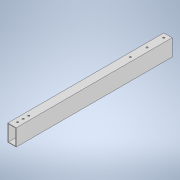
# Autodesk Inventor part: アーム3_角柱1
Saved by Autodesk Inventor 2021 (Build 250183000, 183)
## iProperties
Created: 2022-02-03
Part Number: アーム3_角柱1
Material: 一般
Document SubType Name: Modeling
Designer: hirohumi
Density: 1 g/cm^3
Appearance: 既定
Author: hirohumi
Autodesk Inventor part; units mm, degrees
ref_plane "YZ Plane" through (0, 0, 0) normal (1, 0, 0) x (0, 1, 0)
ref_plane "XZ Plane" through (0, 0, 0) normal (0, 1, 0) x (-1, 0, 0)
ref_plane "XY Plane" through (0, 0, 0) normal (0, 0, 1) x (1, 0, 0)
sketch "スケッチ1" plane through (0, 0, 0) normal (0, 0, 1) x (1, 0, 0)
  line L0 (7.5, 15) -> (-7.5, 15)
  line L1 (-7.5, 15) -> (-7.5, -15)
  line L2 (-7.5, -15) -> (7.5, -15)
  line L3 (7.5, -15) -> (7.5, 15)
  line L4 (7.5, 15) -> (-7.5, -15) construction
  line L5 (-7.5, 15) -> (7.5, -15) construction
  line L6 (-6.5, 14) -> (6.5, 14)
  line L7 (6.5, 14) -> (6.5, -14)
  line L8 (6.5, -14) -> (-6.5, -14)
  line L9 (-6.5, -14) -> (-6.5, 14)
  point P0 (0, 0)
  dimension "d0" = 15
  dimension "d1" = 30
  dimension "d2" = 1
  constraints: 20 end point, 4 parallel, 2 midpoint, 2 perpendicular, 1 horizontal, 3 other
  measures "d0" distance of L2.end L1.end
  measures "d1" distance of L1.end L0.end
  measures "d2" distance between parallel lines of L0 L6
extrude "押し出し1" add sketch "スケッチ1" along normal blind 280
sketch "スケッチ2" plane through (-7.5, 15, 0) normal (0, 1, 0) x (1, 0, 0)
  circle A0 centre (7.5, -7.5) radius 1.6
  circle A1 centre (7.5, -37.5) radius 1.6
  circle A2 centre (7.5, -67.5) radius 1.6
  line L0 (15, 0) -> (0, 0) projected
  circle A3 centre (7.5, -270) radius 1.6
  circle A4 centre (7.5, -260) radius 1.6
  circle A5 centre (7.5, -250) radius 1.6
  line L1 (15, -280) -> (0, -280) projected
  point P0 (7.5, 0)
  point P1 (7.5, 0)
  point P2 (7.5, -280)
  dimension "d5" = 3.2
  dimension "d6" = 3.2
  dimension "d7" = 3.2
  dimension "d8" = 7.5
  dimension "d9" = 30
  dimension "d10" = 30
  dimension "d11" = 3.2
  dimension "d12" = 3.2
  dimension "d13" = 3.2
  dimension "d14" = 10
  dimension "d15" = 10
  dimension "d16" = 10
  constraints: 6 centre point, 6 vertical alignment, 2 midpoint
  measures "d5" diameter of A0
  measures "d6" diameter of A1
  measures "d7" diameter of A2
  measures "d8" distance of point (7.5, 0) A0.centre
  measures "d9" distance of A0.centre A1.centre
  measures "d10" distance of A1.centre A2.centre
  measures "d11" diameter of A3
  measures "d12" diameter of A4
  measures "d13" diameter of A5
  measures "d14" distance of A4.centre A3.centre
  measures "d15" distance of A5.centre A4.centre
  measures "d16" distance from line of L1 A3.centre
extrude "押し出し2" cut sketch "スケッチ2" against normal through all
